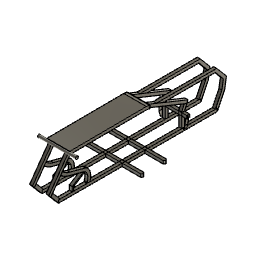
Chassis (Autodesk Fusion 360 design; units mm, degrees)
Autodesk Fusion 360 part; units mm, degrees
sketch "Sketch1" plane through (0, 0, 0) normal (1, 0, 0) x (0, 1, 0) in component "Chassis"
  line L0 (1194, 0) -> (1194, 438.5) construction
  line L1 (1194, 438.5) -> (1194, -438.5) construction
  line L2 (1194, -438.5) -> (-1194, -438.5) construction
  line L3 (1194, 438.5) -> (-1194, 438.5) construction
  line L4 (-1194, 438.5) -> (-1194, -438.5) construction
  line L5 (1194, -438.5) -> (1194, -159.5) construction
  line L6 (1194, -159.5) -> (-1194, -159.5) construction
  line L7 (1194, -438.5) -> (1194, 911.5) construction
  line L8 (1194, 911.5) -> (-1194, 911.5) construction
  line L9 (-1194, 911.5) -> (-1194, -438.5) construction
  dimension "d4" = 438.5
  dimension "d5" = 877
  dimension "d6" = 2388
  dimension "d7" = 2388
  dimension "d8" = 877
  dimension "d9" = 279
  dimension "d11" = 1350
  constraint perpendicular L1 L2
  constraint perpendicular L0 L3
  constraint perpendicular L2 L5
  constraint perpendicular L1 L6
  constraint perpendicular L3 L7
  constraint perpendicular L7 L8
  constraint perpendicular L2 L9
  measures "d4" distance of L0.start L0.end
  measures "d5" distance of L0.end L1.end
  measures "d6" distance of L1.end L2.end
  measures "d7" distance of L0.end L3.end
  measures "d8" distance of L2.end L3.end
  measures "d9" distance of L1.end L5.end
  measures "d11" distance of L1.end L7.end
sketch "Sketch2" plane through (0, 0, 0) normal (1, 0, 0) x (0, 1, 0) in component "Chassis"
  line L0 (1219.0879, -151.0706) -> (-869.559, -151.0706)
  line L1 (1219.0879, -111.0706) -> (-869.559, -111.0706)
  line L2 (1219.0879, -111.0706) -> (1219.0879, -151.0706)
  line L3 (-869.559, -111.0706) -> (-869.559, -151.0706)
  line L4 (819.4204, 140.9941) -> (300, 350)
  line L5 (834.3522, 178.1026) -> (314.9318, 387.1085)
  line L6 (300, 350) -> (314.9318, 387.1085)
  line L7 (819.4204, 140.9941) -> (834.3522, 178.1026)
  line L8 (300, 350) -> (261.9016, 356.1508)
  line L9 (261.9016, 356.1508) -> (-750, 350)
  line L10 (306.3753, 389.4887) -> (264.989, 396.1703)
  line L11 (264.989, 396.1703) -> (-750.2431, 389.9993)
  line L12 (314.9318, 387.1085) -> (306.3753, 389.4887)
  circle A0 centre (-750.1216, 369.9996) radius 20
  line L13 (-750, 350) -> (-997.5729, -0.0699)
  line L14 (-717.3417, 326.9037) -> (-970.8625, -31.5765)
  line L15 (-717.3417, 326.9037) -> (-700.7963, 350.2991)
  arc A1 (-450, -10) -> (-484.2481, 55.6962) centre (-583.5714, -37.8571) ccw
  arc A2 (-455.1421, -111.0706) -> (-450, -10) centre (-645.296, -50.7302) ccw
  arc A3 (-518.1518, 75.4775) -> (-720, 130) centre (-1635.2544, -3659.2663) ccw
  arc A4 (-818.3177, 184.1229) -> (-720, 130) centre (-669.9209, 337.3335) ccw
  arc A5 (-841.646, 151.1366) -> (-729.3915, 91.1181) centre (-669.9209, 337.3335) ccw
  arc A6 (-567.7428, 48.3461) -> (-729.3915, 91.1181) centre (-1635.2544, -3659.2663) ccw
  arc A7 (-489.1575, -18.1665) -> (-500.0447, 10.3611) centre (-583.5714, -37.8571) ccw
  arc A8 (-493.2686, -98.9722) -> (-489.1575, -18.1665) centre (-645.296, -50.7302) ccw
  arc A9 (-497.2694, -111.0706) -> (-493.2686, -98.9722) centre (-995.2398, 60.3154) ccw
  arc A10 (-500.0447, 10.3611) -> (-542.6051, 41.6671) centre (-560.7909, -27.6398) ccw
  arc A11 (-484.2481, 55.6962) -> (-521.4483, 76.462) centre (-545.6531, -10.6025) ccw
  arc A12 (-567.7428, 48.3461) -> (-542.6051, 41.6671) centre (526.6393, 4116.5978) ccw
  line L16 (-869.559, -151.0706) -> (-970.8625, -31.5765)
  line L17 (-851.0299, -111.0706) -> (-940.3514, -5.7101)
  line L18 (-940.3514, -5.7101) -> (-947.0127, 2.1473)
  line L19 (502.0647, 311.8094) -> (1200, 311.8094) construction
  line L20 (414.4973, 347.0451) -> (1212.6349, 347.0451)
  line L21 (513.9051, 307.0451) -> (1194.0535, 307.0451)
  line L22 (-484.2481, 55.6962) -> (1700, 55.6962) construction
  line L23 (1219.0879, -151.0706) -> (1318.3235, 52.4692)
  line L24 (1194.089, -111.0706) -> (1279.737, 64.6)
  line L25 (1279.737, 64.6) -> (1298.3752, 183.4517)
  line L26 (1318.3235, 52.4692) -> (1318.8295, 55.6962)
  line L27 (1298.3752, 183.4517) -> (1200, 300)
  line L28 (1230.0433, -128.6001) -> (1318.3235, 52.4692)
  line L29 (1318.3235, 52.4692) -> (1340.7216, 195.2966)
  line L30 (1340.7216, 195.2966) -> (1230.5668, 325.8006)
  line L31 (1230.5668, 325.8006) -> (1212.6349, 347.0451)
  line L32 (1200, 300) -> (1194.0535, 307.0451)
  line L33 (819.4204, 140.9941) -> (790.8757, 70.055)
  line L34 (790.8757, 70.055) -> (790.8757, -111.0706)
  line L35 (750.8757, 70.055) -> (750.8757, -111.0706)
  line L36 (750.8757, 70.055) -> (750.8757, 77.8009)
  line L37 (782.3119, 155.9259) -> (750.8757, 77.8009)
  line L38 (-671.1178, -111.0706) -> (-671.1178, -50)
  line L39 (-671.1178, -50) -> (-691.1178, -50)
  line L40 (-691.1178, -50) -> (-691.1178, -111.0706)
  line L41 (-691.1178, -50) -> (-542.6051, 41.6671)
  line L42 (-671.1178, -61.1583) -> (-520.6511, 31.7148)
  line L43 (418.2251, 345.5451) -> (1211.9381, 345.5451)
  line L44 (1229.4206, 324.8331) -> (1211.9381, 345.5451)
  line L45 (1299.5214, 184.4192) -> (1201.1463, 300.9675)
  line L46 (1327.7957, 208.2847) -> (1229.4206, 324.8331)
  line L47 (1327.7957, 208.2847) -> (1339.1336, 194.8524)
  line L48 (1201.1463, 300.9675) -> (1194.7503, 308.5451)
  line L49 (513.9051, 308.5451) -> (1194.0535, 308.5451)
  line L50 (1194.0535, 308.5451) -> (1194.7503, 308.5451)
  line L51 (513.9051, 308.5451) -> (510.1773, 308.5451)
  line L52 (818.5888, 142.9456) -> (300.5599, 351.3916)
  line L53 (832.4007, 177.2709) -> (314.3719, 385.7169)
  line L54 (818.5888, 142.9456) -> (832.4007, 177.2709)
  line L55 (818.0288, 141.554) -> (789.3757, 70.3455)
  line L56 (789.3757, 70.3455) -> (789.3757, -111.0706)
  line L57 (783.7035, 155.366) -> (752.3757, 77.5104)
  line L58 (752.3757, 77.5104) -> (752.3757, -111.0706)
  line L59 (1195.4373, -111.728) -> (1281.184, 64.145)
  line L60 (1281.184, 64.145) -> (1299.9632, 183.8959)
  line L61 (1299.9632, 183.8959) -> (1201.1463, 300.9675)
  line L62 (1201.1463, 300.9675) -> (1194.7503, 308.5451)
  line L63 (513.9051, 308.5451) -> (1194.7503, 308.5451)
  line L64 (1228.695, -127.9428) -> (1316.8765, 52.9241)
  line L65 (1316.8765, 52.9241) -> (1336.4103, 177.487)
  line L66 (1336.4103, 177.487) -> (1339.1336, 194.8524)
  line L67 (1228.695, -127.9428) -> (1219.0879, -147.6478)
  line L68 (1217.5879, -149.5706) -> (-867.9119, -149.5706)
  line L69 (1217.5879, -112.5706) -> (1217.5879, -149.5706)
  line L70 (1217.5879, -112.5706) -> (-867.9119, -112.5706)
  line L71 (-869.559, -134.3471) -> (-868.059, -134.3471) construction
  line L72 (-867.9119, -112.5706) -> (-867.9119, -149.5706)
  arc A13 (-456.5718, -110.6169) -> (-451.4684, -10.3062) centre (-645.296, -50.7302) ccw
  arc A14 (-451.4684, -10.3062) -> (-485.3049, 54.6304) centre (-583.5714, -37.8571) ccw
  arc A15 (-485.3049, 54.6304) -> (-521.8501, 75.0168) centre (-545.6531, -10.6025) ccw
  arc A16 (-518.5817, 74.0404) -> (-720.3522, 128.5419) centre (-1635.2544, -3659.2663) ccw
  arc A17 (-819.1941, 182.8837) -> (-720.3522, 128.5419) centre (-669.9209, 337.3335) ccw
  arc A18 (-495.6833, -111.0706) -> (-491.8388, -99.4259) centre (-995.2398, 60.3154) ccw
  arc A19 (-491.8388, -99.4259) -> (-487.6891, -17.8603) centre (-645.296, -50.7302) ccw
  arc A20 (-487.6891, -17.8603) -> (-498.7589, 11.134) centre (-583.5714, -37.8571) ccw
  arc A21 (-498.7589, 11.134) -> (-542.2244, 43.118) centre (-560.7909, -27.6398) ccw
  arc A22 (-567.3405, 49.7912) -> (-542.2244, 43.118) centre (526.6393, 4116.5978) ccw
  arc A23 (-567.3405, 49.7912) -> (-729.0393, 92.5762) centre (-1635.2544, -3659.2663) ccw
  arc A24 (-840.629, 152.2393) -> (-729.0393, 92.5762) centre (-669.9209, 337.3335) ccw
  line L73 (-456.5718, -110.6169) -> (-456.7158, -111.0706)
  line L74 (-840.629, 152.2393) -> (-840.7725, 152.3716)
  line L75 (-688.2619, -50) -> (-541.8172, 40.3907)
  line L76 (-671.1178, -59.3956) -> (-521.439, 32.9912)
  line L77 (-672.6178, -111.0706) -> (-672.6178, -51.5)
  line L78 (-672.6178, -51.5) -> (-689.6178, -51.5)
  line L79 (-689.6178, -51.5) -> (-689.6178, -111.0706)
  line L80 (-672.6178, -111.0706) -> (-672.6178, -109.5706)
  line L81 (-852.9964, -111.0706) -> (-941.4955, -6.6801)
  line L82 (-941.4955, -6.6801) -> (-948.1568, 1.1773)
  line L83 (-869.559, -148.751) -> (-969.7183, -30.6065)
  line L84 (299.0558, 351.6719) -> (262.0174, 357.6515)
  line L85 (262.0174, 357.6515) -> (-742.4099, 351.5462)
  line L86 (306.1362, 388.0079) -> (264.8732, 394.6696)
  line L87 (264.8732, 394.6696) -> (-742.6348, 388.5455)
  line L88 (306.1362, 388.0079) -> (312.9178, 386.1214)
  circle A25 centre (-750.1216, 369.9996) radius 18.5
  line L89 (-718.5664, 327.7699) -> (-970.9698, -29.1304)
  line L90 (-718.5664, 327.7699) -> (-702.6414, 350.2879)
  line L91 (-748.7753, 349.1339) -> (-995.6769, 0.0133)
  line L92 (-748.7753, 349.1339) -> (-748.1549, 350.0112)
  line L93 (-969.7183, -30.6065) -> (-969.9681, -30.3119)
  line L94 (-541.8172, 40.3907) -> (-540.6354, 41.1201)
  line L95 (1508.2935, 585.8008) -> (1508.2935, -430.509)
  line L96 (1508.2935, -430.509) -> (-1200, -430.509)
  line L97 (-1200, -430.509) -> (-1200, 575.8555)
  line L98 (-1200, 575.8555) -> (1508.2935, 585.8008)
  line L99 (299.0558, 351.6719) -> (312.9178, 386.1214)
  line L100 (313.4777, 387.513) -> (313.5403, 387.6684)
  line L101 (-869.559, -151.0706) -> (-997.5729, -0.0699)
  line L102 (-869.559, -148.751) -> (-969.9681, -30.3119)
  line L103 (-970.9698, -29.1304) -> (-995.6769, 0.0133)
  dimension "d17" = 40
  dimension "d18" = 40
  dimension "d19" = 40
  dimension "d27" = 40
  dimension "d29" = 40
  dimension "d31" = 20
  dimension "d35" = 1.5
  dimension "d36" = 38.5
  dimension "d37" = -1.5
  dimension "d41" = 1.5
  dimension "d42" = 38.5
  dimension "d43" = 1.5
  dimension "d44" = 38.5
  dimension "d48" = 1.5
  dimension "d49" = -1.5
  dimension "d54" = -1.5
  dimension "d55" = 1.5
  dimension "d60" = -1.5
  dimension "d127" = 181.1256
  constraint horizontal L0
  constraint perpendicular L0 L2
  constraint perpendicular L0 L3
  constraint coincident L11.end A0
  constraint coincident L9 L15.end
  constraint parallel L14 L15
  constraint parallel L13 L14
  constraint coincident L14 A4.start
  constraint tangent A1 A2
  constraint coincident L1 A2.start
  constraint tangent A3 A4
  constraint tangent A8 A9
  constraint coincident L1 A9.start
  constraint coincident A3 A11.end
  constraint coincident A11 A3.start
  constraint concentric A4 A5
  constraint concentric A3 A6
  constraint concentric A1 A7
  constraint concentric A2 A8
  constraint tangent A5 A6
  constraint tangent A7 A8
  constraint tangent A10 A12
  constraint coincident L14 A5.start
  constraint coincident L14 L18.end
  constraint parallel L17 L18
  constraint parallel L16 L17
  constraint coincident L1 L17.start
  constraint coincident L5 L19.start
  constraint horizontal L19
  constraint coincident L5 L20.start
  constraint horizontal L20
  constraint parallel L20 L21
  constraint coincident L5 L21.start
  constraint horizontal L22
  constraint parallel L23 L24
  constraint coincident L1 L24.start
  constraint parallel L30 L31
  constraint parallel L27 L32
  constraint parallel L25 L26
  constraint perpendicular L4 L33
  constraint coincident L1 L34.end
  constraint perpendicular L1 L34
  constraint parallel L35 L36
  constraint perpendicular L4 L37
  constraint coincident L1 L38.start
  constraint perpendicular L1 L38
  constraint perpendicular L38 L39
  constraint coincident L1 L40.end
  constraint perpendicular L1 L40
  constraint coincident L38 L42.start
  constraint coincident A10 L42.end
  constraint parallel L20 L43
  constraint coincident L5 L43.start
  constraint parallel L46 L47
  constraint parallel L31 L44
  constraint parallel L45 L48
  constraint parallel L49 L50
  constraint coincident L5 L51.end
  constraint parallel L49 L51
  constraint parallel L7 L54
  constraint parallel L4 L53
  constraint parallel L4 L52
  constraint parallel L29 L66
  constraint coincident L2 L67.end
  constraint parallel L64 L67
  constraint coincident L3 L71.start
  constraint horizontal L71
  constraint perpendicular L68 L72
  constraint parallel L0 L68
  constraint parallel L0 L70
  constraint parallel L2 L69
  constraint concentric A9 A18
  constraint concentric A8 A19
  constraint concentric A7 A20
  constraint concentric A10 A21
  constraint concentric A12 A22
  constraint concentric A6 A23
  constraint concentric A5 A24
  constraint tangent A23 A24
  constraint tangent A21 A22
  constraint tangent A19 A20
  constraint tangent A18 A19
  constraint coincident L1 A18.start
  constraint coincident L1 L73.end
  constraint tangent A13 L73
  constraint coincident L14 L74.end
  constraint tangent A24 L74
  constraint concentric A3 A16
  constraint concentric A4 A17
  constraint tangent A16 A17
  constraint coincident L14 A17.start
  constraint parallel L42 L76
  constraint coincident L38 L76.start
  constraint parallel L41 L75
  constraint coincident L39 L75.start
  constraint perpendicular L1 L80
  constraint parallel L8 L86
  constraint parallel L9 L87
  constraint coincident A0 L87.end
  constraint parallel L8 L84
  constraint parallel L9 L85
  constraint coincident A0 L85.end
  constraint parallel L14 L89
  constraint parallel L15 L90
  constraint coincident L9 L90.end
  constraint coincident L9 L92.end
  constraint parallel L13 L91
  constraint coincident L14 L93.end
  constraint parallel L83 L93
  constraint parallel L17 L81
  constraint parallel L18 L82
  constraint coincident L1 L81.start
  constraint parallel L16 L83
  constraint coincident L3 L83.start
  constraint coincident L22 L26.end
  constraint coincident A10 L94.end
  constraint parallel L75 L94
  constraint vertical L95
  constraint perpendicular L95 L96
  constraint perpendicular L96 L97
  constraint parallel L6 L99
  constraint coincident L12 L100.start
  constraint collinear L99 L100
  constraint parallel L16 L102
  constraint parallel L16 L101
  constraint coincident L89.end L102
  constraint collinear L102 L103
  measures "d31" distance of L38.end L39.end
  measures "d48" distance of L71.start L71.end
  measures "d55" distance of L77.start L80.end
  measures "d127" distance of L33.end L34.end
extrude "Extrude1" add sketch "Sketch2" along normal blind -128 and the other way blind 88 contours L0 L1 L2 L3 makes body 1 in component "Chassis"
extrude "Extrude2" add sketch "Sketch2" along normal blind -128 and the other way blind 88 contours L2 L5 L20 L23 L26 L28 L29 L30 L31 L43 L44 L46 L47 L64 L65 L66 L67 | L3 L14 L16 L83 L93 L101 L102 | L9 L13 L14 L15 L89 L90 L91 L92 L101 L103 | L1 L5 L21 L24 L25 L27 L32 L45 L48 L49 L50 L51 L59 L60 L61 L62 L63 | L1 L14 L17 L18 L81 L82 | L1 L4 L33 L34 L55 L56 | L1 L38 L39 L40 L77 L78 L79 L80 | L1 L14 A5 A6 A7 A8 A9 A10 A12 A18 A19 A20 A21 A22 A23 A24 L74 | A10 L39 L41 L75 L94 | L1 L4 L35 L36 L37 L57 L58 | L4 L5 L6 L7 L52 L53 L54 | L1 L14 A1 A2 A3 A4 A11 A13 A14 A15 A16 A17 L73 | A10 L38 L42 L76 | A15 A16 bodies 1 in component "Chassis"
sketch "Sketch4" plane through (0, 0, 0) normal (0, 0, 1) x (1, 0, 0) in component "Chassis"
  line L0 (-127.961, 1362.3849) -> (-127.961, -998.1728)
  line L1 (-126.461, 1362.3849) -> (-126.461, -998.1728)
  line L2 (-87.961, 1362.3849) -> (-87.961, -998.1728)
  line L3 (-89.461, 1362.3849) -> (-89.461, -998.1728)
  line L4 (-127.961, -998.1728) -> (-126.461, -998.1728)
  line L5 (-87.961, -998.1728) -> (-89.461, -998.1728)
  line L6 (-126.461, 1362.3849) -> (-127.961, 1362.3849)
  line L7 (-89.461, 1362.3849) -> (-87.961, 1362.3849)
  dimension "d73" = -40
  dimension "d74" = -38.5
  constraint vertical L0
  constraint perpendicular L1 L4
  constraint parallel L0 L1
  constraint perpendicular L3 L5
  constraint perpendicular L0 L6
  constraint vertical L2
  constraint perpendicular L2 L7
extrude "Extrude3" add sketch "Sketch4" along normal blind 410 and the other way blind 200 bodies 1 in component "Chassis"
extrude "Extrude4" cut sketch "Sketch2" against normal blind 150 contours L1 L5 L7 L21 L24 L25 L27 L32 L33 L34 | L1 L14 A5 A6 A12 L17 L18 L40 L41 | L1 L4 L8 L9 L14 L15 A1 A2 A3 A4 A11 L35 L36 L37 | L1 A7 A8 A9 A10 L38 L42 | A25 | L95 L96 L97 L98 bodies 1 in component "Chassis"
extrude "Extrude5" add sketch "Sketch2" against normal blind 250 contours A0 bodies 1 in component "Chassis"
extrude "Extrude6" add sketch "Sketch2" against normal blind 150 contours L6 L8 L9 L10 L11 L12 A0 L84 L85 L86 L87 L88 L99 bodies 1 in component "Chassis"
extrude "Extrude7" cut sketch "Sketch2" against normal blind 130 contours A0 L84 L85 L86 L87 L88 L99 bodies 1 in component "Chassis"
sketch "Sketch2 (2)" plane through (0, 0, 0) normal (0, 0, 1) x (1, 0, 0)
  line L0 (-150, -750) -> (-150, 315)
  line L1 (-148.5, -750) -> (-148.5, 315)
  line L2 (-148.5, 315) -> (-150, 315)
  line L3 (-148.5, -750) -> (-150, -750)
  dimension "d141" = 1.5
  constraint vertical L0
  constraint perpendicular L0 L2
  constraint perpendicular L0 L3
extrude "Extrude18" add sketch "Sketch2 (2)" along normal blind 397 and the other way blind -350 bodies 1 in component "Chassis"
extrude "Extrude19" cut sketch "Sketch2" against normal blind 600 contours L1 L4 L8 L9 L14 L15 A1 A2 A3 A4 A11 L35 L36 L37 | A25 | L95 L96 L97 L98 bodies 1 in component "Chassis"
sketch "Sketch5" plane through (0, 0, 0) normal (0, 0, 1) x (1, 0, 0) in component "Chassis"
  line L0 (0, 265) -> (-371.0713, 265)
  line L1 (0, 305) -> (-371.0713, 305)
  line L2 (0, 266.5) -> (-370.1909, 266.5)
  line L3 (0, 303.5) -> (-370.1909, 303.5)
  line L4 (-386, 285) -> (-371.0713, 305)
  line L5 (-371.0713, 265) -> (-386, 285)
  line L6 (-370.1909, 266.5) -> (-384, 285)
  line L7 (-384, 285) -> (-370.1909, 303.5)
  line L8 (0, 266.5) -> (0, 265)
  line L9 (0, 303.5) -> (0, 305)
  line L10 (0, -33.5) -> (-374.2297, -33.5)
  line L11 (-390, -15) -> (-375.0713, 5)
  line L12 (0, -33.5) -> (0, -35)
  line L13 (0, 3.5) -> (-374.2297, 3.5)
  line L14 (0, -35) -> (-375.0713, -35)
  line L15 (-388.0387, -15) -> (-374.2297, 3.5)
  line L16 (0, 3.5) -> (0, 5)
  line L17 (0, 5) -> (-375.0713, 5)
  line L18 (-374.2297, -33.5) -> (-388.0387, -15)
  line L19 (-375.0713, -35) -> (-390, -15)
  line L20 (0, 3.5) -> (0, -33.5)
  line L21 (0, 305) -> (0, 265)
  line L22 (0.6449, 39.6025) -> (-250, 39.6025) construction
  line L23 (-384, 285) -> (-384, -50) construction
  dimension "d89" = 40
  dimension "d93" = 40
  dimension "d148" = 250.6449
  constraint horizontal L0
  constraint coincident L1 L4.end
  constraint parallel L5 L6
  constraint parallel L4 L7
  constraint parallel L0 L2
  constraint parallel L0 L3
  constraint perpendicular L0 L8
  constraint perpendicular L1 L9
  constraint horizontal L14
  constraint coincident L11.end L17
  constraint parallel L18 L19
  constraint parallel L11 L15
  constraint parallel L10 L14
  constraint parallel L13 L14
  constraint perpendicular L12 L14
  constraint perpendicular L16 L17
  constraint perpendicular L10 L20
  constraint perpendicular L0 L21
  constraint horizontal L22
  constraint vertical L23
  measures "d148" distance of L22.start L22.end
extrude "Extrude8" add sketch "Sketch5" along normal blind -151.07 and the other way blind 110.2 contours L10 L11 L12 L13 L14 L15 L16 L17 L18 L19 bodies 1 in component "Chassis"
extrude "Extrude9" add sketch "Sketch5" along normal blind -151.07 and the other way blind 149.57 contours L10 L13 L15 L18 L20 bodies 1 in component "Chassis"
extrude "Extrude10" add sketch "Sketch5" along normal blind -111.7 and the other way blind 110.2 contours L10 L13 L15 L18 L20 bodies 1 in component "Chassis"
extrude "Extrude11" add sketch "Sketch5" along normal blind -110.2 and the other way blind 151.07 contours L0 L1 L2 L3 L4 L5 L6 L7 L8 L9 L21 bodies 1 in component "Chassis"
extrude "Extrude12" add sketch "Sketch5" along normal blind -111.7 and the other way blind 110.2 contours L2 L3 L6 L7 L21 bodies 1 in component "Chassis"
extrude "Extrude13" add sketch "Sketch5" along normal blind -151.07 and the other way blind 149.57 contours L2 L3 L6 L7 L21 bodies 1 in component "Chassis"
sketch "Sketch6" plane through (0, 0, 0) normal (0, 1, 0) x (1, 0, 0) in component "Chassis"
  line L0 (-175, 110) -> (-175, 60) construction
  line L1 (-225, 109.8485) -> (-225, -71.2775) construction
  arc A0 (-149.7161, 109.8767) -> (-170.2822, 56.106) centre (-82.1788, 53.2268) ccw
  line L2 (-170.4041, 54.4314) -> (-185.1976, -71.3133)
  arc A1 (-148.3247, 107.2455) -> (-167.5556, 55.2525) centre (-82.1788, 53.2268) ccw
  line L3 (-167.5872, 54.8328) -> (-182.4279, -71.3133)
  line L4 (-148.3247, 107.2455) -> (-146.2016, 109.8452)
  line L5 (-146.2016, 109.8452) -> (-149.7161, 109.8767)
  arc A2 (-170.4041, 54.4314) -> (-170.2822, 56.106) centre (-191.2916, 56.7926) ccw
  arc A3 (-167.5872, 54.8328) -> (-167.5556, 55.2525) centre (-172.5832, 55.4206) ccw
  line L6 (-182.4279, -71.3133) -> (-185.1976, -71.3133)
  dimension "d118" = 50
  dimension "d120" = 181.126
  constraint vertical L0
  constraint vertical L1
  constraint concentric A0 A1
  constraint parallel L2 L3
  constraint tangent A1 L4
  constraint tangent A0 A2
  constraint tangent L3 A3
  constraint horizontal L6
  measures "d118" distance of L0.start L0.end
  measures "d120" distance of L1.start L1.end
extrude "Extrude14" add sketch "Sketch6" along normal blind 791 and the other way blind -751 bodies 1 makes body 2 in component "Chassis"
delete_face "DeleteFace1" 1 faces at (-170.2892, 777.6667, -55.9195) on bodies 2 in component "Chassis"
delete_face "DeleteFace2" 1 faces at (-167.5573, 777.6667, -55.2058) on bodies 2 in component "Chassis"
sketch "Sketch7" plane through (0, 0, 0) normal (1, 0, 0) x (0, 1, 0) in component "Chassis"
  line L0 (751, 71) -> (791, 71)
  line L1 (791, 71) -> (791, 31)
  line L2 (791, 31) -> (751, 31)
  line L3 (751, 31) -> (751, 71)
  line L4 (752.5, 69.5) -> (789.5, 69.5)
  line L5 (789.5, 69.5) -> (789.5, 32.5)
  line L6 (789.5, 32.5) -> (752.5, 32.5)
  line L7 (752.5, 32.5) -> (752.5, 69.5)
  line L8 (750, 72) -> (792, 72)
  line L9 (792, 72) -> (792, 31)
  line L10 (750, 30) -> (750, 72)
  line L11 (751, 31) -> (750, 31)
  line L12 (791, 31) -> (792, 31)
  dimension "d128" = 1.5
  constraint horizontal L0
  constraint perpendicular L0 L1
  constraint perpendicular L1 L2
  constraint perpendicular L0 L3
  constraint coincident L10 L11.end
  constraint perpendicular L10 L11
  constraint parallel L0 L8
  constraint parallel L1 L9
  constraint parallel L3 L10
  constraint perpendicular L9 L12
extrude "Extrude15" add sketch "Sketch7" against normal blind 195 contours L0 L1 L2 L3 bodies 2 1 in component "Chassis"
extrude "Extrude16" cut sketch "Sketch7" against normal blind 420 contours L4 L5 L6 L7 bodies 2 in component "Chassis"
extrude "Extrude17" cut sketch "Sketch7" along normal blind -200 and the other way blind 160 contours L0 L1 L3 L8 L9 L10 L11 L12 bodies 2 in component "Chassis"
mirror "Mirror1" about plane through (0, 0, 0) normal (1, 0, 0) of bodies 2 merged in component "Chassis"
component "Chassis" placed x (1, 0, 0) y (0, 1, 0) z (0, 0, 1) at (0, 0, 0)
